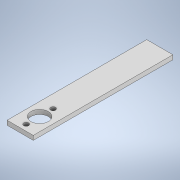
# Autodesk Inventor part: ArmSmall
Saved by Autodesk Inventor 2020 (Build 240168000, 168)
## iProperties
Created: 2020-01-20
Part Number: ArmSmall
Material: Generic
Document SubType Name: Modeling
Designer: tdmp4
Density: 1 g/cm^3
Appearance: Default
Author: tdmp4
Autodesk Inventor part; units mm, degrees
ref_plane "YZ Plane" through (0, 0, 0) normal (1, 0, 0) x (0, 1, 0)
ref_plane "XZ Plane" through (0, 0, 0) normal (0, 1, 0) x (-1, 0, 0)
ref_plane "XY Plane" through (0, 0, 0) normal (0, 0, 1) x (1, 0, 0)
sketch "Sketch1" plane through (0, 0, 0) normal (0, 1, 0) x (-1, 0, 0)
  line L0 (0, 0) -> (19.05, 0)
  line L1 (19.05, 0) -> (19.05, -101.6)
  line L2 (19.05, -101.6) -> (0, -101.6)
  line L3 (0, -101.6) -> (0, 0)
  dimension "d0" = 19.05
  dimension "d1" = 101.6
  constraints: 8 end point, 2 parallel, 1 horizontal, 1 perpendicular
  measures "d0" distance of L1.end L2.end
  measures "d1" distance of L2.end L0.start
extrude "Extrusion1" add sketch "Sketch1" along normal blind 3.175
sketch "Sketch2" plane through (0, 3.175, 0) normal (0, 1, 0) x (1, 0, 0)
  circle A0 centre (-9.525, 14.1659) radius 9.779
  circle A1 centre (-9.525, 4.3869) radius 1.7907
  circle A2 centre (-9.525, 23.9449) radius 1.7907
  circle A3 centre (-9.525, 14.1659) radius 6.35
  point P0 (0, 0)
  dimension "d4" = 19.558
  dimension "d5" = 3.5814
  dimension "d6" = 3.5814
  dimension "d7" = 12.7
  constraints: 4 centre point, 2 point on circle, 1 coincident
  measures "d4" diameter of A0
  measures "d5" diameter of A1
  measures "d6" diameter of A2
  measures "d7" diameter of A3
extrude "Extrusion2" cut sketch "Sketch2" against normal blind 3.175 contours A2 A0 | A0 A2 | A1 A0 | A0 A1 | A3
body "Solid1"
